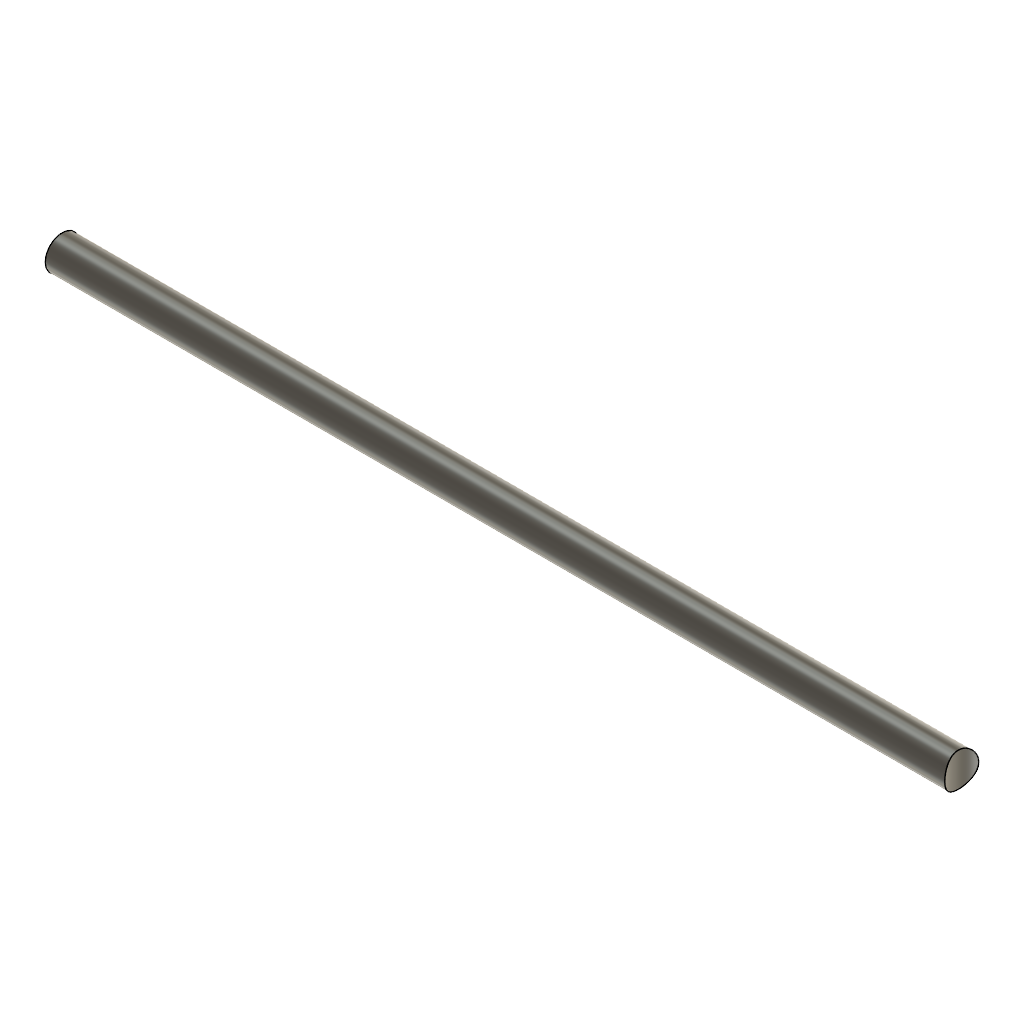
Suspension_Member_V2_Notch_Cutout Model (Autodesk Fusion 360 design; units mm, degrees)
part number: 2026-09-25-22-23-16-836
Autodesk Fusion 360 part; units mm, degrees
sketch "Sketch2" plane through (0, 0, 0) normal (0, 0, 1) x (1, 0, 0)
  line L0 (0, 0) -> (-350, 0)
  line L1 (-350, 0) -> (-350, -6.35)
  line L2 (-350, -6.35) -> (0, -6.35)
  line L3 (0, -6.35) -> (0, 0)
  dimension "d1" = 350
  dimension "d2" = 6.35
  constraint horizontal L0
  constraint vertical L1
  constraint horizontal L2
  constraint vertical L3
  constraint coincident L0.start L3.end
  measures "d1" distance of L0.start L0.end
  measures "d2" distance of L0.start L2.end
revolve "Revolve1" add sketch "Sketch2" angle 360 about axis through (0, 0, 0) along (-1, 0, 0)
sketch "Sketch3" plane through (0, 0, 0) normal (0, 0, 1) x (1, 0, 0)
  circle A0 centre (0, 0) radius 16.25
  dimension "d4" = 32.5
  constraint coincident A0.centre origin
  measures "d4" diameter of A0
extrude "Extrude1" cut sketch "Sketch3" along normal through all and the other way through all
